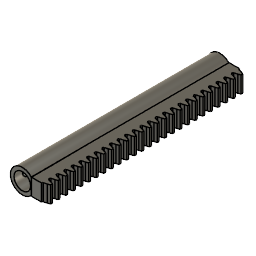
Rack Pen Holder (Autodesk Fusion 360 design; units mm, degrees)
description: Rack; Circular Pitch: 4.12283 mm; Num Teeth: 26; Pressure Angle: 20 deg; Backlash: 0.12 mm;
Autodesk Fusion 360 part; units mm, degrees
note: some values were not read from the file. Set by a fixed rule: which sketch regions a step uses.
(part 1 of 4)
sketch "Sketch1" plane through (0, 0, 0) normal (0, 0, 1) x (1, 0, 0) in component "Rack; Circular Pitch: 4.12283 mm; Num Teeth: 26; Pressure Angle: 20 deg; Backlash: 0.12 mm;"
  line L0 (-1.7283, -1.4496) -> (0, -0.9707)
  line L1 (0, -0.9707) -> (1.3123, -0.4931)
  line L2 (-1.7283, 1.4496) -> (0, 0.9707)
  line L3 (0, 0.9707) -> (1.3123, 0.4931)
  line L4 (1.3123, 0.4931) -> (1.3123, -0.4931)
  line L5 (-2.0948, 1.9315) -> (-2.0948, 2.0614)
  line L6 (-2.0948, -1.9315) -> (-2.0948, -2.0614)
  arc A0 (-2.0948, 1.9315) -> (-1.7283, 1.4496) centre (-1.5948, 1.9315) ccw
  arc A1 (-1.7283, -1.4496) -> (-2.0948, -1.9315) centre (-1.5948, -1.9315) ccw
  line L7 (-1.7283, 2.6732) -> (0, 3.1521)
  line L8 (0, 3.1521) -> (1.3123, 3.6298)
  line L9 (-1.7283, 5.5724) -> (0, 5.0935)
  line L10 (0, 5.0935) -> (1.3123, 4.6159)
  line L11 (1.3123, 4.6159) -> (1.3123, 3.6298)
  line L12 (-2.0948, 6.0543) -> (-2.0948, 6.1842)
  line L13 (-2.0948, 2.1914) -> (-2.0948, 2.0614)
  arc A2 (-2.0948, 6.0543) -> (-1.7283, 5.5724) centre (-1.5948, 6.0543) ccw
  arc A3 (-1.7283, 2.6732) -> (-2.0948, 2.1914) centre (-1.5948, 2.1914) ccw
  line L14 (-1.7283, 6.796) -> (0, 7.275)
  line L15 (0, 7.275) -> (1.3123, 7.7526)
  line L16 (-1.7283, 9.6953) -> (0, 9.2164)
  line L17 (0, 9.2164) -> (1.3123, 8.7387)
  line L18 (1.3123, 8.7387) -> (1.3123, 7.7526)
  line L19 (-2.0948, 10.1771) -> (-2.0948, 10.3071)
  line L20 (-2.0948, 6.3142) -> (-2.0948, 6.1842)
  arc A4 (-2.0948, 10.1771) -> (-1.7283, 9.6953) centre (-1.5948, 10.1771) ccw
  arc A5 (-1.7283, 6.796) -> (-2.0948, 6.3142) centre (-1.5948, 6.3142) ccw
  line L21 (-1.7283, 10.9189) -> (0, 11.3978)
  line L22 (0, 11.3978) -> (1.3123, 11.8754)
  line L23 (-1.7283, 13.8181) -> (0, 13.3392)
  line L24 (0, 13.3392) -> (1.3123, 12.8615)
  line L25 (1.3123, 12.8615) -> (1.3123, 11.8754)
  line L26 (-2.0948, 14.3) -> (-2.0948, 14.4299)
  line L27 (-2.0948, 10.437) -> (-2.0948, 10.3071)
  arc A6 (-2.0948, 14.3) -> (-1.7283, 13.8181) centre (-1.5948, 14.3) ccw
  arc A7 (-1.7283, 10.9189) -> (-2.0948, 10.437) centre (-1.5948, 10.437) ccw
  line L28 (-1.7283, 15.0417) -> (0, 15.5206)
  line L29 (0, 15.5206) -> (1.3123, 15.9983)
  line L30 (-1.7283, 17.9409) -> (0, 17.462)
  line L31 (0, 17.462) -> (1.3123, 16.9844)
  line L32 (1.3123, 16.9844) -> (1.3123, 15.9983)
  line L33 (-2.0948, 18.4228) -> (-2.0948, 18.5527)
  line L34 (-2.0948, 14.5599) -> (-2.0948, 14.4299)
  arc A8 (-2.0948, 18.4228) -> (-1.7283, 17.9409) centre (-1.5948, 18.4228) ccw
  arc A9 (-1.7283, 15.0417) -> (-2.0948, 14.5599) centre (-1.5948, 14.5599) ccw
  line L35 (-1.7283, 19.1645) -> (0, 19.6434)
  line L36 (0, 19.6434) -> (1.3123, 20.1211)
  line L37 (-1.7283, 22.0638) -> (0, 21.5849)
  line L38 (0, 21.5849) -> (1.3123, 21.1072)
  line L39 (1.3123, 21.1072) -> (1.3123, 20.1211)
  line L40 (-2.0948, 22.5456) -> (-2.0948, 22.6756)
  line L41 (-2.0948, 18.6827) -> (-2.0948, 18.5527)
  arc A10 (-2.0948, 22.5456) -> (-1.7283, 22.0638) centre (-1.5948, 22.5456) ccw
  arc A11 (-1.7283, 19.1645) -> (-2.0948, 18.6827) centre (-1.5948, 18.6827) ccw
  line L42 (-1.7283, 23.2874) -> (0, 23.7663)
  line L43 (0, 23.7663) -> (1.3123, 24.2439)
  line L44 (-1.7283, 26.1866) -> (0, 25.7077)
  line L45 (0, 25.7077) -> (1.3123, 25.23)
  line L46 (1.3123, 25.23) -> (1.3123, 24.2439)
  line L47 (-2.0948, 26.6684) -> (-2.0948, 26.7984)
  line L48 (-2.0948, 22.8055) -> (-2.0948, 22.6756)
  arc A12 (-2.0948, 26.6684) -> (-1.7283, 26.1866) centre (-1.5948, 26.6684) ccw
  arc A13 (-1.7283, 23.2874) -> (-2.0948, 22.8055) centre (-1.5948, 22.8055) ccw
  line L49 (-1.7283, 27.4102) -> (0, 27.8891)
  line L50 (0, 27.8891) -> (1.3123, 28.3668)
  line L51 (-1.7283, 30.3094) -> (0, 29.8305)
  line L52 (0, 29.8305) -> (1.3123, 29.3529)
  line L53 (1.3123, 29.3529) -> (1.3123, 28.3668)
  line L54 (-2.0948, 30.7913) -> (-2.0948, 30.9212)
  line L55 (-2.0948, 26.9283) -> (-2.0948, 26.7984)
  arc A14 (-2.0948, 30.7913) -> (-1.7283, 30.3094) centre (-1.5948, 30.7913) ccw
  arc A15 (-1.7283, 27.4102) -> (-2.0948, 26.9283) centre (-1.5948, 26.9283) ccw
  line L56 (-1.7283, 31.533) -> (0, 32.0119)
  line L57 (0, 32.0119) -> (1.3123, 32.4896)
  line L58 (-1.7283, 34.4323) -> (0, 33.9533)
  line L59 (0, 33.9533) -> (1.3123, 33.4757)
  line L60 (1.3123, 33.4757) -> (1.3123, 32.4896)
  line L61 (-2.0948, 34.9141) -> (-2.0948, 35.0441)
  line L62 (-2.0948, 31.0512) -> (-2.0948, 30.9212)
  arc A16 (-2.0948, 34.9141) -> (-1.7283, 34.4323) centre (-1.5948, 34.9141) ccw
  arc A17 (-1.7283, 31.533) -> (-2.0948, 31.0512) centre (-1.5948, 31.0512) ccw
  line L63 (-1.7283, 35.6559) -> (0, 36.1348)
  line L64 (0, 36.1348) -> (1.3123, 36.6124)
  line L65 (-1.7283, 38.5551) -> (0, 38.0762)
  line L66 (0, 38.0762) -> (1.3123, 37.5985)
  line L67 (1.3123, 37.5985) -> (1.3123, 36.6124)
  line L68 (-2.0948, 39.0369) -> (-2.0948, 39.1669)
  line L69 (-2.0948, 35.174) -> (-2.0948, 35.0441)
  arc A18 (-2.0948, 39.0369) -> (-1.7283, 38.5551) centre (-1.5948, 39.0369) ccw
  arc A19 (-1.7283, 35.6559) -> (-2.0948, 35.174) centre (-1.5948, 35.174) ccw
  line L70 (-1.7283, 39.7787) -> (0, 40.2576)
  line L71 (0, 40.2576) -> (1.3123, 40.7352)
  line L72 (-1.7283, 42.6779) -> (0, 42.199)
  line L73 (0, 42.199) -> (1.3123, 41.7214)
  line L74 (1.3123, 41.7214) -> (1.3123, 40.7352)
  line L75 (-2.0948, 43.1598) -> (-2.0948, 43.2897)
  line L76 (-2.0948, 39.2968) -> (-2.0948, 39.1669)
  arc A20 (-2.0948, 43.1598) -> (-1.7283, 42.6779) centre (-1.5948, 43.1598) ccw
  arc A21 (-1.7283, 39.7787) -> (-2.0948, 39.2968) centre (-1.5948, 39.2968) ccw
  line L77 (-1.7283, 43.9015) -> (0, 44.3804)
  line L78 (0, 44.3804) -> (1.3123, 44.8581)
  line L79 (-1.7283, 46.8007) -> (0, 46.3218)
  line L80 (0, 46.3218) -> (1.3123, 45.8442)
  line L81 (1.3123, 45.8442) -> (1.3123, 44.8581)
  line L82 (-2.0948, 47.2826) -> (-2.0948, 47.4125)
  line L83 (-2.0948, 43.4197) -> (-2.0948, 43.2897)
  arc A22 (-2.0948, 47.2826) -> (-1.7283, 46.8007) centre (-1.5948, 47.2826) ccw
  arc A23 (-1.7283, 43.9015) -> (-2.0948, 43.4197) centre (-1.5948, 43.4197) ccw
  line L84 (-1.7283, 48.0243) -> (0, 48.5033)
  line L85 (0, 48.5033) -> (1.3123, 48.9809)
  line L86 (-1.7283, 50.9236) -> (0, 50.4447)
  line L87 (0, 50.4447) -> (1.3123, 49.967)
  line L88 (1.3123, 49.967) -> (1.3123, 48.9809)
  line L89 (-2.0948, 51.4054) -> (-2.0948, 51.5354)
  line L90 (-2.0948, 47.5425) -> (-2.0948, 47.4125)
  arc A24 (-2.0948, 51.4054) -> (-1.7283, 50.9236) centre (-1.5948, 51.4054) ccw
  arc A25 (-1.7283, 48.0243) -> (-2.0948, 47.5425) centre (-1.5948, 47.5425) ccw
  line L91 (-1.7283, 52.1472) -> (0, 52.6261)
  line L92 (0, 52.6261) -> (1.3123, 53.1037)
  line L93 (-1.7283, 55.0464) -> (0, 54.5675)
  line L94 (0, 54.5675) -> (1.3123, 54.0898)
  line L95 (1.3123, 54.0898) -> (1.3123, 53.1037)
  line L96 (-2.0948, 55.5283) -> (-2.0948, 55.6582)
  line L97 (-2.0948, 51.6653) -> (-2.0948, 51.5354)
  arc A26 (-2.0948, 55.5283) -> (-1.7283, 55.0464) centre (-1.5948, 55.5283) ccw
  arc A27 (-1.7283, 52.1472) -> (-2.0948, 51.6653) centre (-1.5948, 51.6653) ccw
  line L98 (-1.7283, 56.27) -> (0, 56.7489)
  line L99 (0, 56.7489) -> (1.3123, 57.2266)
  line L100 (-1.7283, 59.1692) -> (0, 58.6903)
  line L101 (0, 58.6903) -> (1.3123, 58.2127)
  line L102 (1.3123, 58.2127) -> (1.3123, 57.2266)
  line L103 (-2.0948, 59.6511) -> (-2.0948, 59.781)
  line L104 (-2.0948, 55.7882) -> (-2.0948, 55.6582)
  arc A28 (-2.0948, 59.6511) -> (-1.7283, 59.1692) centre (-1.5948, 59.6511) ccw
  arc A29 (-1.7283, 56.27) -> (-2.0948, 55.7882) centre (-1.5948, 55.7882) ccw
  line L105 (-1.7283, 60.3928) -> (0, 60.8717)
  line L106 (0, 60.8717) -> (1.3123, 61.3494)
  line L107 (-1.7283, 63.2921) -> (0, 62.8132)
  line L108 (0, 62.8132) -> (1.3123, 62.3355)
  line L109 (1.3123, 62.3355) -> (1.3123, 61.3494)
  line L110 (-2.0948, 63.7739) -> (-2.0948, 63.9039)
  line L111 (-2.0948, 59.911) -> (-2.0948, 59.781)
  arc A30 (-2.0948, 63.7739) -> (-1.7283, 63.2921) centre (-1.5948, 63.7739) ccw
  arc A31 (-1.7283, 60.3928) -> (-2.0948, 59.911) centre (-1.5948, 59.911) ccw
  line L112 (-1.7283, 64.5157) -> (0, 64.9946)
  line L113 (0, 64.9946) -> (1.3123, 65.4722)
  line L114 (-1.7283, 67.4149) -> (0, 66.936)
  line L115 (0, 66.936) -> (1.3123, 66.4583)
  line L116 (1.3123, 66.4583) -> (1.3123, 65.4722)
  line L117 (-2.0948, 67.8967) -> (-2.0948, 68.0267)
  line L118 (-2.0948, 64.0338) -> (-2.0948, 63.9039)
  arc A32 (-2.0948, 67.8967) -> (-1.7283, 67.4149) centre (-1.5948, 67.8967) ccw
  arc A33 (-1.7283, 64.5157) -> (-2.0948, 64.0338) centre (-1.5948, 64.0338) ccw
  line L119 (-1.7283, 68.6385) -> (0, 69.1174)
  line L120 (0, 69.1174) -> (1.3123, 69.5951)
  line L121 (-1.7283, 71.5377) -> (0, 71.0588)
  line L122 (0, 71.0588) -> (1.3123, 70.5812)
  line L123 (1.3123, 70.5812) -> (1.3123, 69.5951)
  line L124 (-2.0948, 72.0196) -> (-2.0948, 72.1495)
  line L125 (-2.0948, 68.1566) -> (-2.0948, 68.0267)
  arc A34 (-2.0948, 72.0196) -> (-1.7283, 71.5377) centre (-1.5948, 72.0196) ccw
  arc A35 (-1.7283, 68.6385) -> (-2.0948, 68.1566) centre (-1.5948, 68.1566) ccw
  line L126 (-1.7283, 72.7613) -> (0, 73.2402)
  line L127 (0, 73.2402) -> (1.3123, 73.7179)
  line L128 (-1.7283, 75.6606) -> (0, 75.1816)
  line L129 (0, 75.1816) -> (1.3123, 74.704)
  line L130 (1.3123, 74.704) -> (1.3123, 73.7179)
  line L131 (-2.0948, 76.1424) -> (-2.0948, 76.2724)
  line L132 (-2.0948, 72.2795) -> (-2.0948, 72.1495)
  arc A36 (-2.0948, 76.1424) -> (-1.7283, 75.6606) centre (-1.5948, 76.1424) ccw
  arc A37 (-1.7283, 72.7613) -> (-2.0948, 72.2795) centre (-1.5948, 72.2795) ccw
  line L133 (-1.7283, 76.8842) -> (0, 77.3631)
  line L134 (0, 77.3631) -> (1.3123, 77.8407)
  line L135 (-1.7283, 79.7834) -> (0, 79.3045)
  line L136 (0, 79.3045) -> (1.3123, 78.8268)
  line L137 (1.3123, 78.8268) -> (1.3123, 77.8407)
  line L138 (-2.0948, 80.2652) -> (-2.0948, 80.3952)
  line L139 (-2.0948, 76.4023) -> (-2.0948, 76.2724)
  arc A38 (-2.0948, 80.2652) -> (-1.7283, 79.7834) centre (-1.5948, 80.2652) ccw
  arc A39 (-1.7283, 76.8842) -> (-2.0948, 76.4023) centre (-1.5948, 76.4023) ccw
  line L140 (-1.7283, 81.007) -> (0, 81.4859)
  line L141 (0, 81.4859) -> (1.3123, 81.9635)
  line L142 (-1.7283, 83.9062) -> (0, 83.4273)
  line L143 (0, 83.4273) -> (1.3123, 82.9497)
  line L144 (1.3123, 82.9497) -> (1.3123, 81.9635)
  line L145 (-2.0948, 84.3881) -> (-2.0948, 84.518)
  line L146 (-2.0948, 80.5251) -> (-2.0948, 80.3952)
  arc A40 (-2.0948, 84.3881) -> (-1.7283, 83.9062) centre (-1.5948, 84.3881) ccw
  arc A41 (-1.7283, 81.007) -> (-2.0948, 80.5251) centre (-1.5948, 80.5251) ccw
  line L147 (-1.7283, 85.1298) -> (0, 85.6087)
  line L148 (0, 85.6087) -> (1.3123, 86.0864)
  line L149 (-1.7283, 88.029) -> (0, 87.5501)
  line L150 (0, 87.5501) -> (1.3123, 87.0725)
  line L151 (1.3123, 87.0725) -> (1.3123, 86.0864)
  line L152 (-2.0948, 88.5109) -> (-2.0948, 88.6408)
  line L153 (-2.0948, 84.648) -> (-2.0948, 84.518)
  arc A42 (-2.0948, 88.5109) -> (-1.7283, 88.029) centre (-1.5948, 88.5109) ccw
  arc A43 (-1.7283, 85.1298) -> (-2.0948, 84.648) centre (-1.5948, 84.648) ccw
  line L154 (-1.7283, 89.2526) -> (0, 89.7316)
  line L155 (0, 89.7316) -> (1.3123, 90.2092)
  line L156 (-1.7283, 92.1519) -> (0, 91.673)
  line L157 (0, 91.673) -> (1.3123, 91.1953)
  line L158 (1.3123, 91.1953) -> (1.3123, 90.2092)
  line L159 (-2.0948, 92.6337) -> (-2.0948, 92.7637)
  line L160 (-2.0948, 88.7708) -> (-2.0948, 88.6408)
  arc A44 (-2.0948, 92.6337) -> (-1.7283, 92.1519) centre (-1.5948, 92.6337) ccw
  arc A45 (-1.7283, 89.2526) -> (-2.0948, 88.7708) centre (-1.5948, 88.7708) ccw
  line L161 (-1.7283, 93.3755) -> (0, 93.8544)
  line L162 (0, 93.8544) -> (1.3123, 94.332)
  line L163 (-1.7283, 96.2747) -> (0, 95.7958)
  line L164 (0, 95.7958) -> (1.3123, 95.3181)
  line L165 (1.3123, 95.3181) -> (1.3123, 94.332)
  line L166 (-2.0948, 96.7566) -> (-2.0948, 96.8865)
  line L167 (-2.0948, 92.8936) -> (-2.0948, 92.7637)
  arc A46 (-2.0948, 96.7566) -> (-1.7283, 96.2747) centre (-1.5948, 96.7566) ccw
  arc A47 (-1.7283, 93.3755) -> (-2.0948, 92.8936) centre (-1.5948, 92.8936) ccw
  line L168 (-1.7283, 97.4983) -> (0, 97.9772)
  line L169 (0, 97.9772) -> (1.3123, 98.4549)
  line L170 (-1.7283, 100.3975) -> (0, 99.9186)
  line L171 (0, 99.9186) -> (1.3123, 99.441)
  line L172 (1.3123, 99.441) -> (1.3123, 98.4549)
  line L173 (-2.0948, 100.8794) -> (-2.0948, 101.0093)
  line L174 (-2.0948, 97.0165) -> (-2.0948, 96.8865)
  arc A48 (-2.0948, 100.8794) -> (-1.7283, 100.3975) centre (-1.5948, 100.8794) ccw
  arc A49 (-1.7283, 97.4983) -> (-2.0948, 97.0165) centre (-1.5948, 97.0165) ccw
  line L175 (-1.7283, 101.6211) -> (0, 102.1)
  line L176 (0, 102.1) -> (1.3123, 102.5777)
  line L177 (-1.7283, 104.5204) -> (0, 104.0415)
  line L178 (0, 104.0415) -> (1.3123, 103.5638)
  line L179 (1.3123, 103.5638) -> (1.3123, 102.5777)
  line L180 (-2.0948, 105.0022) -> (-2.0948, 105.1322)
  line L181 (-2.0948, 101.1393) -> (-2.0948, 101.0093)
  arc A50 (-2.0948, 105.0022) -> (-1.7283, 104.5204) centre (-1.5948, 105.0022) ccw
  arc A51 (-1.7283, 101.6211) -> (-2.0948, 101.1393) centre (-1.5948, 101.1393) ccw
  line L182 (-1.7283, 105.744) -> (0, 106.2229)
  line L183 (0, 106.2229) -> (1.3123, 106.7005)
  line L184 (-1.7283, 108.6432) -> (0, 108.1643)
  line L185 (0, 108.1643) -> (1.3123, 107.6866)
  line L186 (1.3123, 107.6866) -> (1.3123, 106.7005)
  line L187 (-2.0948, 109.125) -> (-2.0948, 109.255)
  line L188 (-2.0948, 105.2621) -> (-2.0948, 105.1322)
  arc A52 (-2.0948, 109.125) -> (-1.7283, 108.6432) centre (-1.5948, 109.125) ccw
  arc A53 (-1.7283, 105.744) -> (-2.0948, 105.2621) centre (-1.5948, 105.2621) ccw
  line L189 (-2.0948, -2.0614) -> (-7.5948, -2.0614)
  line L190 (-7.5948, -2.0614) -> (-8.0948, 105.1322)
  line L191 (-8.0948, 105.1322) -> (-2.0948, 105.1322)
  constraint tangent L2 A0
  constraint tangent L5 A0
  constraint tangent L0 A1
  constraint tangent L6 A1
  constraint tangent L9 A2
  constraint tangent L12 A2
  constraint tangent L7 A3
  constraint tangent L13 A3
  constraint tangent L16 A4
  constraint tangent L19 A4
  constraint tangent L14 A5
  constraint tangent L20 A5
  constraint tangent L23 A6
  constraint tangent L26 A6
  constraint tangent L21 A7
  constraint tangent L27 A7
  constraint tangent L30 A8
  constraint tangent L33 A8
  constraint tangent L28 A9
  constraint tangent L34 A9
  constraint tangent L37 A10
  constraint tangent L40 A10
  constraint tangent L35 A11
  constraint tangent L41 A11
  constraint tangent L44 A12
  constraint tangent L47 A12
  constraint tangent L42 A13
  constraint tangent L48 A13
  constraint tangent L51 A14
  constraint tangent L54 A14
  constraint tangent L49 A15
  constraint tangent L55 A15
  constraint tangent L58 A16
  constraint tangent L61 A16
  constraint tangent L56 A17
  constraint tangent L62 A17
  constraint tangent L65 A18
  constraint tangent L68 A18
  constraint tangent L63 A19
  constraint tangent L69 A19
  constraint tangent L72 A20
  constraint tangent L75 A20
  constraint tangent L70 A21
  constraint tangent L76 A21
  constraint tangent L79 A22
  constraint tangent L82 A22
  constraint tangent L77 A23
  constraint tangent L83 A23
  constraint tangent L86 A24
  constraint tangent L89 A24
  constraint tangent L84 A25
  constraint tangent L90 A25
  constraint tangent L93 A26
  constraint tangent L96 A26
  constraint tangent L91 A27
  constraint tangent L97 A27
  constraint tangent L100 A28
  constraint tangent L103 A28
  constraint tangent L98 A29
  constraint tangent L104 A29
  constraint tangent L107 A30
  constraint tangent L110 A30
  constraint tangent L105 A31
  constraint tangent L111 A31
  constraint tangent L114 A32
  constraint tangent L117 A32
  constraint tangent L112 A33
  constraint tangent L118 A33
  constraint tangent L121 A34
  constraint tangent L124 A34
  constraint tangent L119 A35
  constraint tangent L125 A35
  constraint tangent L128 A36
  constraint tangent L131 A36
  constraint tangent L126 A37
  constraint tangent L132 A37
  constraint tangent L135 A38
  constraint tangent L138 A38
  constraint tangent L133 A39
  constraint tangent L139 A39
  constraint tangent L142 A40
  constraint tangent L145 A40
  constraint tangent L140 A41
  constraint tangent L146 A41
  constraint tangent L149 A42
  constraint tangent L152 A42
  constraint tangent L147 A43
  constraint tangent L153 A43
  constraint tangent L156 A44
  constraint tangent L159 A44
  constraint tangent L154 A45
  constraint tangent L160 A45
  constraint tangent L163 A46
  constraint tangent L166 A46
  constraint tangent L161 A47
  constraint tangent L167 A47
  constraint tangent L170 A48
  constraint tangent L173 A48
  constraint tangent L168 A49
  constraint tangent L174 A49
  constraint tangent L177 A50
  constraint tangent L180 A50
  constraint tangent L175 A51
  constraint tangent L181 A51
  constraint tangent L184 A52
  constraint tangent L187 A52
  constraint tangent L182 A53
  constraint tangent L188 A53
extrude "Extrude1" add sketch "Sketch1" along normal blind 4.5 and the other way blind 4.5 makes body 1 in component "Rack; Circular Pitch: 4.12283 mm; Num Teeth: 26; Pressure Angle: 20 deg; Backlash: 0.12 mm;"
sketch "Sketch2" plane through (0, 0, 0) normal (0, 0, 1) x (1, 0, 0) in component "Rack; Circular Pitch: 4.12283 mm; Num Teeth: 26; Pressure Angle: 20 deg; Backlash: 0.12 mm;"
  line L0 (0, 0) -> (0, 103.0708) construction
sketch "Sketch1 (2)" plane through (0, 0, 8) normal (0, 0, 1) x (-1, 0, 0)
  arc A0 (-32.6491, -24.8397) -> (-32.7083, -25.327) centre (-17.3506, -26.9445) ccw
  arc A1 (-33.2417, -25.7733) -> (-32.7083, -25.327) centre (-33.2055, -25.2746) ccw
  line L0 (-33.2417, -25.7733) -> (-33.3469, -25.7656)
  spline S0 degree 5 poles (-33.3469, -25.7656) (-33.3537, -25.7652) (-33.3673, -25.7643) (-33.3878, -25.7636) (-33.4151, -25.7635) (-33.4493, -25.7648) (-33.4836, -25.7669) (-33.5178, -25.7697) (-33.5521, -25.7728) (-33.5864, -25.7761) (-33.6207, -25.7796) (-33.655, -25.7834) (-33.6893, -25.7876) (-33.7236, -25.7922) (-33.7579, -25.7974) (-33.7922, -25.8029) (-33.8265, -25.8088) (-33.8609, -25.815) (-33.8952, -25.8214) (-33.9295, -25.8282) (-33.9638, -25.8351) (-33.9981, -25.8424) (-34.0324, -25.8499) (-34.0667, -25.8577) (-34.101, -25.8657) (-34.1353, -25.8741) (-34.1695, -25.8827) (-34.2038, -25.8915) (-34.238, -25.9006) (-34.2723, -25.9099) (-34.3065, -25.9194) (-34.3407, -25.9292) (-34.3749, -25.9392) (-34.4091, -25.9494) (-34.4433, -25.9599) (-34.4775, -25.9706) (-34.5116, -25.9815) (-34.5457, -25.9926) (-34.5799, -26.0039) (-34.614, -26.0154) (-34.6481, -26.0271) (-34.6821, -26.0391) (-34.7162, -26.0512) (-34.7502, -26.0635) (-34.7842, -26.0761) (-34.8182, -26.0888) (-34.8522, -26.1017) (-34.8861, -26.1149) (-34.9201, -26.1282) (-34.954, -26.1417) (-34.9879, -26.1554) (-35.0218, -26.1692) (-35.0556, -26.1833) (-35.0894, -26.1976) (-35.1232, -26.212) (-35.157, -26.2266) (-35.1908, -26.2414) (-35.2245, -26.2564) (-35.2582, -26.2715) (-35.2919, -26.2868) (-35.3256, -26.3023) (-35.3592, -26.318) (-35.3928, -26.3339) (-35.4264, -26.3499) (-35.4599, -26.3661) (-35.4934, -26.3824) (-35.5269, -26.399) (-35.5604, -26.4157) (-35.5938, -26.4325) (-35.6272, -26.4495) (-35.6606, -26.4667) (-35.6873, -26.4806) (-35.7073, -26.4911) (-35.7206, -26.4981) (-35.7273, -26.5017) knots 0 0 0 0 0 0 0.01428571 0.02857143 0.04285714 0.05714286 0.07142857 0.08571429 0.1 0.11428571 0.12857143 0.14285714 0.15714286 0.17142857 0.18571429 0.2 0.21428571 0.22857143 0.24285714 0.25714286 0.27142857 0.28571429 0.3 0.31428571 0.32857143 0.34285714 0.35714286 0.37142857 0.38571429 0.4 0.41428571 0.42857143 0.44285714 0.45714286 0.47142857 0.48571429 0.5 0.51428571 0.52857143 0.54285714 0.55714286 0.57142857 0.58571429 0.6 0.61428571 0.62857143 0.64285714 0.65714286 0.67142857 0.68571429 0.7 0.71428571 0.72857143 0.74285714 0.75714286 0.77142857 0.78571429 0.8 0.81428571 0.82857143 0.84285714 0.85714286 0.87142857 0.88571429 0.9 0.91428571 0.92857143 0.94285714 0.95714286 0.97142857 0.98571429 1 1 1 1 1 1
  arc A2 (-35.7273, -26.5017) -> (-35.7273, -27.3873) centre (-17.3506, -26.9445) ccw
  spline S1 degree 5 poles (-35.7273, -27.3873) (-35.7206, -27.3908) (-35.7073, -27.3979) (-35.6873, -27.4084) (-35.6606, -27.4222) (-35.6272, -27.4394) (-35.5938, -27.4565) (-35.5604, -27.4733) (-35.5269, -27.49) (-35.4934, -27.5066) (-35.4599, -27.5229) (-35.4264, -27.5391) (-35.3928, -27.5551) (-35.3592, -27.571) (-35.3256, -27.5866) (-35.2919, -27.6021) (-35.2582, -27.6175) (-35.2245, -27.6326) (-35.1908, -27.6476) (-35.157, -27.6624) (-35.1232, -27.677) (-35.0894, -27.6914) (-35.0556, -27.7057) (-35.0218, -27.7197) (-34.9879, -27.7336) (-34.954, -27.7473) (-34.9201, -27.7608) (-34.8861, -27.7741) (-34.8522, -27.7872) (-34.8182, -27.8002) (-34.7842, -27.8129) (-34.7502, -27.8254) (-34.7162, -27.8378) (-34.6821, -27.8499) (-34.6481, -27.8618) (-34.614, -27.8736) (-34.5799, -27.8851) (-34.5457, -27.8964) (-34.5116, -27.9075) (-34.4775, -27.9184) (-34.4433, -27.9291) (-34.4091, -27.9395) (-34.3749, -27.9498) (-34.3407, -27.9598) (-34.3065, -27.9695) (-34.2723, -27.9791) (-34.238, -27.9884) (-34.2038, -27.9975) (-34.1695, -28.0063) (-34.1353, -28.0149) (-34.101, -28.0233) (-34.0667, -28.0313) (-34.0324, -28.0391) (-33.9981, -28.0466) (-33.9638, -28.0538) (-33.9295, -28.0608) (-33.8952, -28.0675) (-33.8609, -28.074) (-33.8265, -28.0802) (-33.7922, -28.0861) (-33.7579, -28.0916) (-33.7236, -28.0967) (-33.6893, -28.1014) (-33.655, -28.1056) (-33.6207, -28.1094) (-33.5864, -28.1129) (-33.5521, -28.1162) (-33.5178, -28.1193) (-33.4836, -28.1221) (-33.4493, -28.1242) (-33.4151, -28.1254) (-33.3878, -28.1254) (-33.3673, -28.1247) (-33.3537, -28.1238) (-33.3469, -28.1233) knots -1 -1 -1 -1 -1 -1 -0.98571429 -0.97142857 -0.95714286 -0.94285714 -0.92857143 -0.91428571 -0.9 -0.88571429 -0.87142857 -0.85714286 -0.84285714 -0.82857143 -0.81428571 -0.8 -0.78571429 -0.77142857 -0.75714286 -0.74285714 -0.72857143 -0.71428571 -0.7 -0.68571429 -0.67142857 -0.65714286 -0.64285714 -0.62857143 -0.61428571 -0.6 -0.58571429 -0.57142857 -0.55714286 -0.54285714 -0.52857143 -0.51428571 -0.5 -0.48571429 -0.47142857 -0.45714286 -0.44285714 -0.42857143 -0.41428571 -0.4 -0.38571429 -0.37142857 -0.35714286 -0.34285714 -0.32857143 -0.31428571 -0.3 -0.28571429 -0.27142857 -0.25714286 -0.24285714 -0.22857143 -0.21428571 -0.2 -0.18571429 -0.17142857 -0.15714286 -0.14285714 -0.12857143 -0.11428571 -0.1 -0.08571429 -0.07142857 -0.05714286 -0.04285714 -0.02857143 -0.01428571 0 0 0 0 0 0
  line L1 (-33.3469, -28.1233) -> (-33.2417, -28.1157)
  arc A3 (-32.7083, -28.562) -> (-33.2417, -28.1157) centre (-33.2055, -28.6144) ccw
  arc A4 (-32.7083, -28.562) -> (-32.6491, -29.0493) centre (-17.3506, -26.9445) ccw
  arc A5 (-33.0602, -29.6103) -> (-32.6491, -29.0493) centre (-33.1444, -29.1174) ccw
  line L2 (-33.0602, -29.6103) -> (-33.1641, -29.6281)
  spline S2 degree 5 poles (-33.1641, -29.6281) (-33.1709, -29.6292) (-33.1843, -29.6317) (-33.2044, -29.6358) (-33.231, -29.6423) (-33.2639, -29.6517) (-33.2966, -29.662) (-33.3292, -29.6729) (-33.3617, -29.6841) (-33.3942, -29.6955) (-33.4267, -29.7071) (-33.4591, -29.719) (-33.4914, -29.7313) (-33.5236, -29.744) (-33.5557, -29.7572) (-33.5877, -29.7708) (-33.6196, -29.7847) (-33.6514, -29.799) (-33.6832, -29.8135) (-33.7149, -29.8282) (-33.7465, -29.8432) (-33.7781, -29.8584) (-33.8096, -29.8739) (-33.8411, -29.8897) (-33.8724, -29.9057) (-33.9037, -29.922) (-33.9349, -29.9386) (-33.9661, -29.9553) (-33.9971, -29.9724) (-34.0282, -29.9896) (-34.0591, -30.007) (-34.09, -30.0247) (-34.1208, -30.0426) (-34.1516, -30.0607) (-34.1822, -30.0791) (-34.2129, -30.0976) (-34.2434, -30.1163) (-34.2739, -30.1353) (-34.3043, -30.1544) (-34.3347, -30.1738) (-34.365, -30.1933) (-34.3952, -30.2131) (-34.4253, -30.233) (-34.4554, -30.2531) (-34.4855, -30.2734) (-34.5154, -30.2939) (-34.5453, -30.3146) (-34.5751, -30.3355) (-34.6049, -30.3565) (-34.6346, -30.3778) (-34.6642, -30.3992) (-34.6938, -30.4208) (-34.7233, -30.4425) (-34.7527, -30.4644) (-34.7821, -30.4865) (-34.8114, -30.5088) (-34.8406, -30.5313) (-34.8698, -30.5539) (-34.8989, -30.5766) (-34.9279, -30.5996) (-34.9569, -30.6227) (-34.9858, -30.6459) (-35.0147, -30.6694) (-35.0434, -30.693) (-35.0721, -30.7167) (-35.1008, -30.7406) (-35.1293, -30.7647) (-35.1578, -30.7889) (-35.1862, -30.8133) (-35.2146, -30.8378) (-35.2429, -30.8625) (-35.2655, -30.8824) (-35.2824, -30.8973) (-35.2936, -30.9073) (-35.2993, -30.9124) knots 0 0 0 0 0 0 0.01428571 0.02857143 0.04285714 0.05714286 0.07142857 0.08571429 0.1 0.11428571 0.12857143 0.14285714 0.15714286 0.17142857 0.18571429 0.2 0.21428571 0.22857143 0.24285714 0.25714286 0.27142857 0.28571429 0.3 0.31428571 0.32857143 0.34285714 0.35714286 0.37142857 0.38571429 0.4 0.41428571 0.42857143 0.44285714 0.45714286 0.47142857 0.48571429 0.5 0.51428571 0.52857143 0.54285714 0.55714286 0.57142857 0.58571429 0.6 0.61428571 0.62857143 0.64285714 0.65714286 0.67142857 0.68571429 0.7 0.71428571 0.72857143 0.74285714 0.75714286 0.77142857 0.78571429 0.8 0.81428571 0.82857143 0.84285714 0.85714286 0.87142857 0.88571429 0.9 0.91428571 0.92857143 0.94285714 0.95714286 0.97142857 0.98571429 1 1 1 1 1 1
  arc A6 (-35.2993, -30.9124) -> (-35.0873, -31.7723) centre (-17.3506, -26.9445) ccw
  spline S3 degree 5 poles (-35.0873, -31.7723) (-35.08, -31.7741) (-35.0654, -31.7777) (-35.0435, -31.7831) (-35.0142, -31.7902) (-34.9777, -31.7989) (-34.9412, -31.8075) (-34.9047, -31.8158) (-34.8682, -31.824) (-34.8317, -31.8321) (-34.7953, -31.8399) (-34.7588, -31.8476) (-34.7224, -31.8552) (-34.686, -31.8625) (-34.6496, -31.8697) (-34.6132, -31.8767) (-34.5768, -31.8835) (-34.5404, -31.8901) (-34.5041, -31.8966) (-34.4678, -31.9029) (-34.4315, -31.909) (-34.3952, -31.9149) (-34.359, -31.9206) (-34.3227, -31.9262) (-34.2865, -31.9316) (-34.2504, -31.9367) (-34.2142, -31.9417) (-34.1781, -31.9465) (-34.1419, -31.9512) (-34.1059, -31.9556) (-34.0698, -31.9598) (-34.0338, -31.9638) (-33.9978, -31.9677) (-33.9618, -31.9713) (-33.9259, -31.9747) (-33.89, -31.978) (-33.8541, -31.981) (-33.8183, -31.9838) (-33.7825, -31.9864) (-33.7467, -31.9888) (-33.711, -31.991) (-33.6753, -31.993) (-33.6397, -31.9947) (-33.6041, -31.9963) (-33.5685, -31.9976) (-33.533, -31.9986) (-33.4975, -31.9995) (-33.4621, -32.0001) (-33.4267, -32.0005) (-33.3914, -32.0006) (-33.3561, -32.0005) (-33.3209, -32.0002) (-33.2857, -31.9995) (-33.2506, -31.9986) (-33.2156, -31.9974) (-33.1806, -31.996) (-33.1457, -31.9943) (-33.1108, -31.9923) (-33.076, -31.9902) (-33.0413, -31.9877) (-33.0066, -31.9848) (-32.9721, -31.9816) (-32.9376, -31.9779) (-32.9033, -31.9737) (-32.8691, -31.9692) (-32.835, -31.9644) (-32.8009, -31.9594) (-32.7669, -31.9542) (-32.733, -31.9487) (-32.6992, -31.9426) (-32.6657, -31.9356) (-32.6392, -31.929) (-32.6195, -31.9234) (-32.6064, -31.9193) (-32.5999, -31.9172) knots -1 -1 -1 -1 -1 -1 -0.98571429 -0.97142857 -0.95714286 -0.94285714 -0.92857143 -0.91428571 -0.9 -0.88571429 -0.87142857 -0.85714286 -0.84285714 -0.82857143 -0.81428571 -0.8 -0.78571429 -0.77142857 -0.75714286 -0.74285714 -0.72857143 -0.71428571 -0.7 -0.68571429 -0.67142857 -0.65714286 -0.64285714 -0.62857143 -0.61428571 -0.6 -0.58571429 -0.57142857 -0.55714286 -0.54285714 -0.52857143 -0.51428571 -0.5 -0.48571429 -0.47142857 -0.45714286 -0.44285714 -0.42857143 -0.41428571 -0.4 -0.38571429 -0.37142857 -0.35714286 -0.34285714 -0.32857143 -0.31428571 -0.3 -0.28571429 -0.27142857 -0.25714286 -0.24285714 -0.22857143 -0.21428571 -0.2 -0.18571429 -0.17142857 -0.15714286 -0.14285714 -0.12857143 -0.11428571 -0.1 -0.08571429 -0.07142857 -0.05714286 -0.04285714 -0.02857143 -0.01428571 0 0 0 0 0 0
  line L3 (-32.5999, -31.9172) -> (-32.4996, -31.8847)
  arc A7 (-31.8749, -32.1904) -> (-32.4996, -31.8847) centre (-32.3452, -32.3602) ccw
  arc A8 (-31.8749, -32.1904) -> (-31.7009, -32.6493) centre (-17.3506, -26.9445) ccw
  arc A9 (-31.9657, -33.2924) -> (-31.7009, -32.6493) centre (-32.1655, -32.834) ccw
  line L4 (-31.9657, -33.2924) -> (-32.0624, -33.3345)
  spline S4 degree 5 poles (-32.0624, -33.3345) (-32.0687, -33.3372) (-32.0812, -33.3428) (-32.0996, -33.3517) (-32.1239, -33.3644) (-32.1536, -33.3813) (-32.1829, -33.3992) (-32.2119, -33.4175) (-32.2408, -33.4362) (-32.2697, -33.455) (-32.2984, -33.4741) (-32.327, -33.4934) (-32.3554, -33.5131) (-32.3836, -33.5331) (-32.4117, -33.5536) (-32.4395, -33.5744) (-32.4671, -33.5956) (-32.4946, -33.617) (-32.522, -33.6387) (-32.5493, -33.6606) (-32.5764, -33.6827) (-32.6034, -33.7051) (-32.6303, -33.7277) (-32.657, -33.7505) (-32.6837, -33.7736) (-32.7101, -33.7969) (-32.7365, -33.8204) (-32.7627, -33.8442) (-32.7888, -33.8681) (-32.8148, -33.8923) (-32.8407, -33.9167) (-32.8664, -33.9412) (-32.8921, -33.966) (-32.9176, -33.9909) (-32.943, -34.016) (-32.9683, -34.0414) (-32.9935, -34.0669) (-33.0185, -34.0926) (-33.0435, -34.1185) (-33.0683, -34.1445) (-33.0931, -34.1707) (-33.1177, -34.1971) (-33.1422, -34.2237) (-33.1666, -34.2504) (-33.1909, -34.2773) (-33.2151, -34.3044) (-33.2391, -34.3317) (-33.2631, -34.3591) (-33.287, -34.3866) (-33.3107, -34.4143) (-33.3344, -34.4422) (-33.3579, -34.4702) (-33.3814, -34.4984) (-33.4047, -34.5268) (-33.4279, -34.5552) (-33.451, -34.5839) (-33.474, -34.6127) (-33.497, -34.6416) (-33.5198, -34.6707) (-33.5425, -34.6999) (-33.5651, -34.7293) (-33.5876, -34.7588) (-33.6099, -34.7884) (-33.6322, -34.8182) (-33.6544, -34.8481) (-33.6765, -34.8782) (-33.6985, -34.9084) (-33.7203, -34.9387) (-33.7421, -34.9692) (-33.7638, -34.9998) (-33.7853, -35.0305) (-33.8025, -35.0552) (-33.8153, -35.0738) (-33.8239, -35.0862) (-33.8281, -35.0924) knots 0 0 0 0 0 0 0.01428571 0.02857143 0.04285714 0.05714286 0.07142857 0.08571429 0.1 0.11428571 0.12857143 0.14285714 0.15714286 0.17142857 0.18571429 0.2 0.21428571 0.22857143 0.24285714 0.25714286 0.27142857 0.28571429 0.3 0.31428571 0.32857143 0.34285714 0.35714286 0.37142857 0.38571429 0.4 0.41428571 0.42857143 0.44285714 0.45714286 0.47142857 0.48571429 0.5 0.51428571 0.52857143 0.54285714 0.55714286 0.57142857 0.58571429 0.6 0.61428571 0.62857143 0.64285714 0.65714286 0.67142857 0.68571429 0.7 0.71428571 0.72857143 0.74285714 0.75714286 0.77142857 0.78571429 0.8 0.81428571 0.82857143 0.84285714 0.85714286 0.87142857 0.88571429 0.9 0.91428571 0.92857143 0.94285714 0.95714286 0.97142857 0.98571429 1 1 1 1 1 1
  arc A10 (-33.8281, -35.0924) -> (-33.4166, -35.8767) centre (-17.3506, -26.9445) ccw
  spline S5 degree 5 poles (-33.4166, -35.8767) (-33.409, -35.8767) (-33.394, -35.8767) (-33.3714, -35.8767) (-33.3413, -35.8766) (-33.3038, -35.8763) (-33.2663, -35.8759) (-33.2288, -35.8753) (-33.1914, -35.8745) (-33.1541, -35.8736) (-33.1168, -35.8725) (-33.0796, -35.8712) (-33.0424, -35.8698) (-33.0053, -35.8682) (-32.9682, -35.8665) (-32.9312, -35.8645) (-32.8943, -35.8625) (-32.8574, -35.8602) (-32.8206, -35.8578) (-32.7838, -35.8552) (-32.7471, -35.8524) (-32.7104, -35.8495) (-32.6739, -35.8464) (-32.6374, -35.8431) (-32.6009, -35.8397) (-32.5646, -35.836) (-32.5282, -35.8322) (-32.492, -35.8283) (-32.4558, -35.8241) (-32.4198, -35.8198) (-32.3837, -35.8152) (-32.3478, -35.8105) (-32.3119, -35.8056) (-32.2761, -35.8006) (-32.2404, -35.7953) (-32.2048, -35.7898) (-32.1692, -35.7842) (-32.1338, -35.7783) (-32.0984, -35.7723) (-32.0631, -35.7661) (-32.0279, -35.7597) (-31.9928, -35.753) (-31.9577, -35.7462) (-31.9228, -35.7392) (-31.888, -35.7319) (-31.8532, -35.7245) (-31.8186, -35.7168) (-31.784, -35.7089) (-31.7496, -35.7008) (-31.7152, -35.6925) (-31.681, -35.684) (-31.6469, -35.6752) (-31.6129, -35.6661) (-31.5791, -35.6568) (-31.5453, -35.6473) (-31.5117, -35.6375) (-31.4782, -35.6275) (-31.4448, -35.6173) (-31.4115, -35.6069) (-31.3784, -35.5961) (-31.3455, -35.5851) (-31.3127, -35.5736) (-31.2802, -35.5618) (-31.2478, -35.5496) (-31.2157, -35.537) (-31.1837, -35.5242) (-31.1518, -35.5112) (-31.12, -35.498) (-31.0884, -35.4845) (-31.0571, -35.4705) (-31.0262, -35.4557) (-31.002, -35.443) (-30.9843, -35.4328) (-30.9726, -35.4257) (-30.9667, -35.4221) knots -1 -1 -1 -1 -1 -1 -0.98571429 -0.97142857 -0.95714286 -0.94285714 -0.92857143 -0.91428571 -0.9 -0.88571429 -0.87142857 -0.85714286 -0.84285714 -0.82857143 -0.81428571 -0.8 -0.78571429 -0.77142857 -0.75714286 -0.74285714 -0.72857143 -0.71428571 -0.7 -0.68571429 -0.67142857 -0.65714286 -0.64285714 -0.62857143 -0.61428571 -0.6 -0.58571429 -0.57142857 -0.55714286 -0.54285714 -0.52857143 -0.51428571 -0.5 -0.48571429 -0.47142857 -0.45714286 -0.44285714 -0.42857143 -0.41428571 -0.4 -0.38571429 -0.37142857 -0.35714286 -0.34285714 -0.32857143 -0.31428571 -0.3 -0.28571429 -0.27142857 -0.25714286 -0.24285714 -0.22857143 -0.21428571 -0.2 -0.18571429 -0.17142857 -0.15714286 -0.14285714 -0.12857143 -0.11428571 -0.1 -0.08571429 -0.07142857 -0.05714286 -0.04285714 -0.02857143 -0.01428571 0 0 0 0 0 0
  line L5 (-30.9667, -35.4221) -> (-30.8771, -35.3665)
  arc A11 (-30.1974, -35.5138) -> (-30.8771, -35.3665) centre (-30.6134, -35.7913) ccw
  arc A12 (-30.1974, -35.5138) -> (-29.9186, -35.9178) centre (-17.3506, -26.9445) ccw
  arc A13 (-30.0219, -36.6055) -> (-29.9186, -35.9178) centre (-30.3255, -36.2083) ccw
  line L6 (-30.0219, -36.6055) -> (-30.1057, -36.6696)
  spline S6 degree 5 poles (-30.1057, -36.6696) (-30.1111, -36.6737) (-30.1219, -36.6822) (-30.1377, -36.6952) (-30.1582, -36.7133) (-30.183, -36.7369) (-30.2072, -36.7612) (-30.231, -36.786) (-30.2546, -36.811) (-30.2781, -36.8362) (-30.3014, -36.8616) (-30.3245, -36.8872) (-30.3474, -36.9131) (-30.37, -36.9393) (-30.3923, -36.9659) (-30.4144, -36.9928) (-30.4361, -37.02) (-30.4577, -37.0474) (-30.4791, -37.075) (-30.5003, -37.1027) (-30.5214, -37.1307) (-30.5423, -37.1589) (-30.563, -37.1872) (-30.5835, -37.2158) (-30.6038, -37.2446) (-30.6239, -37.2735) (-30.6439, -37.3027) (-30.6637, -37.332) (-30.6833, -37.3616) (-30.7027, -37.3912) (-30.722, -37.4211) (-30.7411, -37.4511) (-30.7601, -37.4812) (-30.7789, -37.5116) (-30.7976, -37.5421) (-30.8161, -37.5727) (-30.8344, -37.6035) (-30.8526, -37.6344) (-30.8706, -37.6655) (-30.8885, -37.6968) (-30.9063, -37.7282) (-30.9238, -37.7597) (-30.9413, -37.7913) (-30.9586, -37.8232) (-30.9757, -37.8551) (-30.9927, -37.8872) (-31.0096, -37.9194) (-31.0263, -37.9517) (-31.0429, -37.9842) (-31.0593, -38.0168) (-31.0756, -38.0495) (-31.0917, -38.0823) (-31.1078, -38.1153) (-31.1236, -38.1484) (-31.1394, -38.1816) (-31.155, -38.215) (-31.1704, -38.2484) (-31.1857, -38.282) (-31.2009, -38.3157) (-31.216, -38.3495) (-31.2309, -38.3834) (-31.2457, -38.4175) (-31.2603, -38.4516) (-31.2748, -38.4859) (-31.2892, -38.5202) (-31.3034, -38.5547) (-31.3175, -38.5893) (-31.3315, -38.624) (-31.3454, -38.6588) (-31.3591, -38.6937) (-31.3727, -38.7287) (-31.3834, -38.7568) (-31.3914, -38.7779) (-31.3967, -38.792) (-31.3994, -38.799) knots 0 0 0 0 0 0 0.01428571 0.02857143 0.04285714 0.05714286 0.07142857 0.08571429 0.1 0.11428571 0.12857143 0.14285714 0.15714286 0.17142857 0.18571429 0.2 0.21428571 0.22857143 0.24285714 0.25714286 0.27142857 0.28571429 0.3 0.31428571 0.32857143 0.34285714 0.35714286 0.37142857 0.38571429 0.4 0.41428571 0.42857143 0.44285714 0.45714286 0.47142857 0.48571429 0.5 0.51428571 0.52857143 0.54285714 0.55714286 0.57142857 0.58571429 0.6 0.61428571 0.62857143 0.64285714 0.65714286 0.67142857 0.68571429 0.7 0.71428571 0.72857143 0.74285714 0.75714286 0.77142857 0.78571429 0.8 0.81428571 0.82857143 0.84285714 0.85714286 0.87142857 0.88571429 0.9 0.91428571 0.92857143 0.94285714 0.95714286 0.97142857 0.98571429 1 1 1 1 1 1
  arc A14 (-31.3994, -38.799) -> (-30.8121, -39.4619) centre (-17.3506, -26.9445) ccw
  spline S7 degree 5 poles (-30.8121, -39.4619) (-30.8048, -39.4602) (-30.7901, -39.4566) (-30.7682, -39.4512) (-30.739, -39.4439) (-30.7027, -39.4346) (-30.6664, -39.4252) (-30.6302, -39.4156) (-30.594, -39.406) (-30.558, -39.3961) (-30.5221, -39.3861) (-30.4862, -39.376) (-30.4505, -39.3657) (-30.4148, -39.3553) (-30.3792, -39.3447) (-30.3438, -39.334) (-30.3084, -39.3232) (-30.2731, -39.3121) (-30.2379, -39.301) (-30.2029, -39.2897) (-30.1679, -39.2782) (-30.133, -39.2666) (-30.0982, -39.2548) (-30.0636, -39.2429) (-30.029, -39.2308) (-29.9946, -39.2186) (-29.9602, -39.2062) (-29.926, -39.1937) (-29.8919, -39.181) (-29.8579, -39.1681) (-29.824, -39.1551) (-29.7902, -39.142) (-29.7566, -39.1286) (-29.723, -39.1151) (-29.6896, -39.1015) (-29.6563, -39.0876) (-29.6232, -39.0736) (-29.5901, -39.0595) (-29.5572, -39.0452) (-29.5244, -39.0307) (-29.4918, -39.016) (-29.4593, -39.0012) (-29.4269, -38.9862) (-29.3946, -38.971) (-29.3626, -38.9556) (-29.3306, -38.94) (-29.2988, -38.9243) (-29.2671, -38.9084) (-29.2356, -38.8923) (-29.2043, -38.876) (-29.1731, -38.8595) (-29.1421, -38.8428) (-29.1112, -38.8259) (-29.0806, -38.8088) (-29.0501, -38.7914) (-29.0198, -38.7739) (-28.9897, -38.7562) (-28.9597, -38.7383) (-28.9299, -38.7201) (-28.9003, -38.7018) (-28.871, -38.6832) (-28.8419, -38.6642) (-28.8131, -38.645) (-28.7847, -38.6254) (-28.7564, -38.6055) (-28.7284, -38.5854) (-28.7006, -38.5651) (-28.6729, -38.5447) (-28.6454, -38.524) (-28.6184, -38.503) (-28.592, -38.4812) (-28.5715, -38.463) (-28.5567, -38.4489) (-28.547, -38.4392) (-28.5423, -38.4343) knots -1 -1 -1 -1 -1 -1 -0.98571429 -0.97142857 -0.95714286 -0.94285714 -0.92857143 -0.91428571 -0.9 -0.88571429 -0.87142857 -0.85714286 -0.84285714 -0.82857143 -0.81428571 -0.8 -0.78571429 -0.77142857 -0.75714286 -0.74285714 -0.72857143 -0.71428571 -0.7 -0.68571429 -0.67142857 -0.65714286 -0.64285714 -0.62857143 -0.61428571 -0.6 -0.58571429 -0.57142857 -0.55714286 -0.54285714 -0.52857143 -0.51428571 -0.5 -0.48571429 -0.47142857 -0.45714286 -0.44285714 -0.42857143 -0.41428571 -0.4 -0.38571429 -0.37142857 -0.35714286 -0.34285714 -0.32857143 -0.31428571 -0.3 -0.28571429 -0.27142857 -0.25714286 -0.24285714 -0.22857143 -0.21428571 -0.2 -0.18571429 -0.17142857 -0.15714286 -0.14285714 -0.12857143 -0.11428571 -0.1 -0.08571429 -0.07142857 -0.05714286 -0.04285714 -0.02857143 -0.01428571 0 0 0 0 0 0
  line L7 (-28.5423, -38.4343) -> (-28.4686, -38.3589)
  arc A15 (-27.7734, -38.3392) -> (-28.4686, -38.3589) centre (-28.1108, -38.7082) ccw
  arc A16 (-27.7734, -38.3392) -> (-27.406, -38.6647) centre (-17.3506, -26.9445) ccw
  arc A17 (-27.3417, -39.3572) -> (-27.406, -38.6647) centre (-27.7315, -39.0442) ccw
  line L8 (-27.3417, -39.3572) -> (-27.4077, -39.4395)
  spline S8 degree 5 poles (-27.4077, -39.4395) (-27.412, -39.4448) (-27.4204, -39.4556) (-27.4326, -39.472) (-27.4482, -39.4945) (-27.4666, -39.5233) (-27.4843, -39.5527) (-27.5015, -39.5825) (-27.5184, -39.6124) (-27.5352, -39.6425) (-27.5518, -39.6727) (-27.5681, -39.7031) (-27.5841, -39.7338) (-27.5998, -39.7646) (-27.6151, -39.7958) (-27.63, -39.8272) (-27.6447, -39.8588) (-27.6591, -39.8905) (-27.6732, -39.9224) (-27.6872, -39.9545) (-27.701, -39.9867) (-27.7145, -40.019) (-27.7278, -40.0515) (-27.7409, -40.0842) (-27.7537, -40.117) (-27.7663, -40.1499) (-27.7787, -40.183) (-27.7909, -40.2162) (-27.8029, -40.2496) (-27.8147, -40.283) (-27.8263, -40.3166) (-27.8377, -40.3503) (-27.8489, -40.3842) (-27.8599, -40.4181) (-27.8707, -40.4522) (-27.8813, -40.4864) (-27.8917, -40.5206) (-27.902, -40.555) (-27.9121, -40.5896) (-27.9219, -40.6242) (-27.9317, -40.6589) (-27.9412, -40.6937) (-27.9505, -40.7286) (-27.9597, -40.7636) (-27.9687, -40.7987) (-27.9776, -40.834) (-27.9862, -40.8693) (-27.9947, -40.9047) (-28.003, -40.9402) (-28.0112, -40.9757) (-28.0192, -41.0114) (-28.027, -41.0472) (-28.0346, -41.083) (-28.0421, -41.1189) (-28.0495, -41.155) (-28.0566, -41.1911) (-28.0636, -41.2272) (-28.0705, -41.2635) (-28.0771, -41.2999) (-28.0837, -41.3363) (-28.09, -41.3728) (-28.0962, -41.4094) (-28.1023, -41.446) (-28.1082, -41.4828) (-28.1139, -41.5196) (-28.1195, -41.5565) (-28.1249, -41.5934) (-28.1302, -41.6304) (-28.1353, -41.6675) (-28.1403, -41.7047) (-28.1451, -41.7419) (-28.1488, -41.7718) (-28.1515, -41.7942) (-28.1533, -41.8092) (-28.1542, -41.8166) knots 0 0 0 0 0 0 0.01428571 0.02857143 0.04285714 0.05714286 0.07142857 0.08571429 0.1 0.11428571 0.12857143 0.14285714 0.15714286 0.17142857 0.18571429 0.2 0.21428571 0.22857143 0.24285714 0.25714286 0.27142857 0.28571429 0.3 0.31428571 0.32857143 0.34285714 0.35714286 0.37142857 0.38571429 0.4 0.41428571 0.42857143 0.44285714 0.45714286 0.47142857 0.48571429 0.5 0.51428571 0.52857143 0.54285714 0.55714286 0.57142857 0.58571429 0.6 0.61428571 0.62857143 0.64285714 0.65714286 0.67142857 0.68571429 0.7 0.71428571 0.72857143 0.74285714 0.75714286 0.77142857 0.78571429 0.8 0.81428571 0.82857143 0.84285714 0.85714286 0.87142857 0.88571429 0.9 0.91428571 0.92857143 0.94285714 0.95714286 0.97142857 0.98571429 1 1 1 1 1 1
  arc A18 (-28.1542, -41.8166) -> (-27.4253, -42.3197) centre (-17.3506, -26.9445) ccw
  spline S9 degree 5 poles (-27.4253, -42.3197) (-27.4186, -42.3163) (-27.4053, -42.3093) (-27.3853, -42.2988) (-27.3587, -42.2847) (-27.3256, -42.267) (-27.2926, -42.2492) (-27.2597, -42.2313) (-27.227, -42.2132) (-27.1943, -42.195) (-27.1618, -42.1767) (-27.1295, -42.1583) (-27.0972, -42.1398) (-27.0651, -42.1211) (-27.0331, -42.1024) (-27.0012, -42.0835) (-26.9694, -42.0645) (-26.9378, -42.0453) (-26.9063, -42.0261) (-26.875, -42.0067) (-26.8438, -41.9872) (-26.8127, -41.9676) (-26.7818, -41.9478) (-26.751, -41.9279) (-26.7203, -41.908) (-26.6898, -41.8878) (-26.6594, -41.8676) (-26.6292, -41.8472) (-26.5991, -41.8267) (-26.5691, -41.8061) (-26.5393, -41.7854) (-26.5097, -41.7645) (-26.4802, -41.7435) (-26.4509, -41.7224) (-26.4217, -41.7011) (-26.3927, -41.6797) (-26.3638, -41.6582) (-26.3351, -41.6366) (-26.3066, -41.6148) (-26.2783, -41.5929) (-26.2501, -41.5708) (-26.222, -41.5486) (-26.1942, -41.5263) (-26.1665, -41.5038) (-26.1391, -41.4812) (-26.1118, -41.4585) (-26.0847, -41.4356) (-26.0577, -41.4125) (-26.031, -41.3894) (-26.0044, -41.366) (-25.9781, -41.3426) (-25.952, -41.3189) (-25.9261, -41.2951) (-25.9004, -41.2712) (-25.875, -41.2471) (-25.8498, -41.2228) (-25.8248, -41.1984) (-25.7999, -41.1738) (-25.7753, -41.1491) (-25.751, -41.1242) (-25.7269, -41.0991) (-25.7033, -41.0737) (-25.6799, -41.0481) (-25.657, -41.0223) (-25.6344, -40.9962) (-25.612, -40.97) (-25.5898, -40.9437) (-25.5678, -40.9172) (-25.5461, -40.8906) (-25.5248, -40.8636) (-25.5044, -40.8362) (-25.4889, -40.8137) (-25.4779, -40.7964) (-25.4708, -40.7847) (-25.4673, -40.7788) knots -1 -1 -1 -1 -1 -1 -0.98571429 -0.97142857 -0.95714286 -0.94285714 -0.92857143 -0.91428571 -0.9 -0.88571429 -0.87142857 -0.85714286 -0.84285714 -0.82857143 -0.81428571 -0.8 -0.78571429 -0.77142857 -0.75714286 -0.74285714 -0.72857143 -0.71428571 -0.7 -0.68571429 -0.67142857 -0.65714286 -0.64285714 -0.62857143 -0.61428571 -0.6 -0.58571429 -0.57142857 -0.55714286 -0.54285714 -0.52857143 -0.51428571 -0.5 -0.48571429 -0.47142857 -0.45714286 -0.44285714 -0.42857143 -0.41428571 -0.4 -0.38571429 -0.37142857 -0.35714286 -0.34285714 -0.32857143 -0.31428571 -0.3 -0.28571429 -0.27142857 -0.25714286 -0.24285714 -0.22857143 -0.21428571 -0.2 -0.18571429 -0.17142857 -0.15714286 -0.14285714 -0.12857143 -0.11428571 -0.1 -0.08571429 -0.07142857 -0.05714286 -0.04285714 -0.02857143 -0.01428571 0 0 0 0 0 0
  line L9 (-25.4673, -40.7788) -> (-25.4139, -40.6879)
  arc A19 (-24.7436, -40.5025) -> (-25.4139, -40.6879) centre (-24.9829, -40.9414) ccw
  arc A20 (-24.7436, -40.5025) -> (-24.3089, -40.7306) centre (-17.3506, -26.9445) ccw
  arc A21 (-24.0808, -41.3876) -> (-24.3089, -40.7306) centre (-24.5342, -41.1769) ccw
  line L10 (-24.0808, -41.3876) -> (-24.1252, -41.4832)
  spline S10 degree 5 poles (-24.1252, -41.4832) (-24.1281, -41.4894) (-24.1337, -41.5019) (-24.1416, -41.5208) (-24.1514, -41.5463) (-24.1624, -41.5787) (-24.1725, -41.6115) (-24.1821, -41.6445) (-24.1913, -41.6776) (-24.2004, -41.7108) (-24.2093, -41.7442) (-24.2179, -41.7776) (-24.2261, -41.8112) (-24.2339, -41.8449) (-24.2413, -41.8788) (-24.2483, -41.9128) (-24.255, -41.947) (-24.2613, -41.9813) (-24.2675, -42.0157) (-24.2734, -42.0502) (-24.279, -42.0847) (-24.2844, -42.1193) (-24.2896, -42.1541) (-24.2944, -42.1889) (-24.299, -42.2238) (-24.3034, -42.2588) (-24.3075, -42.2939) (-24.3114, -42.3291) (-24.315, -42.3643) (-24.3185, -42.3996) (-24.3217, -42.435) (-24.3247, -42.4705) (-24.3275, -42.506) (-24.33, -42.5416) (-24.3324, -42.5773) (-24.3345, -42.613) (-24.3364, -42.6488) (-24.3382, -42.6847) (-24.3397, -42.7206) (-24.341, -42.7565) (-24.3421, -42.7926) (-24.343, -42.8287) (-24.3438, -42.8648) (-24.3443, -42.901) (-24.3446, -42.9372) (-24.3448, -42.9735) (-24.3447, -43.0099) (-24.3445, -43.0463) (-24.3441, -43.0828) (-24.3435, -43.1193) (-24.3427, -43.1558) (-24.3418, -43.1924) (-24.3406, -43.229) (-24.3393, -43.2657) (-24.3378, -43.3024) (-24.3361, -43.3392) (-24.3342, -43.376) (-24.3322, -43.4129) (-24.33, -43.4497) (-24.3276, -43.4867) (-24.325, -43.5236) (-24.3223, -43.5606) (-24.3194, -43.5977) (-24.3163, -43.6348) (-24.3131, -43.6719) (-24.3097, -43.709) (-24.3061, -43.7462) (-24.3024, -43.7834) (-24.2985, -43.8206) (-24.2944, -43.8579) (-24.2901, -43.8952) (-24.2866, -43.9251) (-24.2839, -43.9475) (-24.2821, -43.9625) (-24.2811, -43.9699) knots 0 0 0 0 0 0 0.01428571 0.02857143 0.04285714 0.05714286 0.07142857 0.08571429 0.1 0.11428571 0.12857143 0.14285714 0.15714286 0.17142857 0.18571429 0.2 0.21428571 0.22857143 0.24285714 0.25714286 0.27142857 0.28571429 0.3 0.31428571 0.32857143 0.34285714 0.35714286 0.37142857 0.38571429 0.4 0.41428571 0.42857143 0.44285714 0.45714286 0.47142857 0.48571429 0.5 0.51428571 0.52857143 0.54285714 0.55714286 0.57142857 0.58571429 0.6 0.61428571 0.62857143 0.64285714 0.65714286 0.67142857 0.68571429 0.7 0.71428571 0.72857143 0.74285714 0.75714286 0.77142857 0.78571429 0.8 0.81428571 0.82857143 0.84285714 0.85714286 0.87142857 0.88571429 0.9 0.91428571 0.92857143 0.94285714 0.95714286 0.97142857 0.98571429 1 1 1 1 1 1
  arc A22 (-24.2811, -43.9699) -> (-23.453, -44.284) centre (-17.3506, -26.9445) ccw
  spline S11 degree 5 poles (-23.453, -44.284) (-23.4474, -44.279) (-23.4361, -44.2691) (-23.4192, -44.2541) (-23.3967, -44.2341) (-23.3688, -44.2089) (-23.341, -44.1837) (-23.3134, -44.1585) (-23.2859, -44.1331) (-23.2586, -44.1076) (-23.2314, -44.0821) (-23.2044, -44.0565) (-23.1775, -44.0307) (-23.1508, -44.0049) (-23.1242, -43.9791) (-23.0978, -43.9531) (-23.0715, -43.927) (-23.0454, -43.9009) (-23.0194, -43.8747) (-22.9936, -43.8483) (-22.968, -43.8219) (-22.9425, -43.7954) (-22.9172, -43.7689) (-22.892, -43.7422) (-22.867, -43.7155) (-22.8422, -43.6886) (-22.8176, -43.6617) (-22.7931, -43.6347) (-22.7688, -43.6076) (-22.7446, -43.5804) (-22.7207, -43.5531) (-22.6969, -43.5258) (-22.6733, -43.4983) (-22.6499, -43.4708) (-22.6266, -43.4432) (-22.6036, -43.4155) (-22.5807, -43.3877) (-22.558, -43.3598) (-22.5355, -43.3318) (-22.5132, -43.3037) (-22.4912, -43.2756) (-22.4693, -43.2473) (-22.4476, -43.219) (-22.4261, -43.1905) (-22.4048, -43.162) (-22.3838, -43.1334) (-22.3629, -43.1047) (-22.3423, -43.0759) (-22.3219, -43.047) (-22.3017, -43.018) (-22.2817, -42.9889) (-22.262, -42.9597) (-22.2426, -42.9304) (-22.2234, -42.901) (-22.2045, -42.8715) (-22.1858, -42.8419) (-22.1673, -42.8122) (-22.1491, -42.7824) (-22.1312, -42.7525) (-22.1135, -42.7225) (-22.0961, -42.6924) (-22.0792, -42.6621) (-22.0627, -42.6316) (-22.0466, -42.6011) (-22.0308, -42.5703) (-22.0154, -42.5395) (-22.0001, -42.5086) (-21.9851, -42.4777) (-21.9704, -42.4466) (-21.9562, -42.4154) (-21.943, -42.3838) (-21.9333, -42.3583) (-21.9267, -42.3389) (-21.9227, -42.3258) (-21.9207, -42.3193) knots -1 -1 -1 -1 -1 -1 -0.98571429 -0.97142857 -0.95714286 -0.94285714 -0.92857143 -0.91428571 -0.9 -0.88571429 -0.87142857 -0.85714286 -0.84285714 -0.82857143 -0.81428571 -0.8 -0.78571429 -0.77142857 -0.75714286 -0.74285714 -0.72857143 -0.71428571 -0.7 -0.68571429 -0.67142857 -0.65714286 -0.64285714 -0.62857143 -0.61428571 -0.6 -0.58571429 -0.57142857 -0.55714286 -0.54285714 -0.52857143 -0.51428571 -0.5 -0.48571429 -0.47142857 -0.45714286 -0.44285714 -0.42857143 -0.41428571 -0.4 -0.38571429 -0.37142857 -0.35714286 -0.34285714 -0.32857143 -0.31428571 -0.3 -0.28571429 -0.27142857 -0.25714286 -0.24285714 -0.22857143 -0.21428571 -0.2 -0.18571429 -0.17142857 -0.15714286 -0.14285714 -0.12857143 -0.11428571 -0.1 -0.08571429 -0.07142857 -0.05714286 -0.04285714 -0.02857143 -0.01428571 0 0 0 0 0 0
  line L11 (-21.9207, -42.3193) -> (-21.8906, -42.2182)
  arc A23 (-21.2841, -41.8777) -> (-21.8906, -42.2182) centre (-21.4115, -42.3612) ccw
  arc A24 (-21.2841, -41.8777) -> (-20.8075, -41.9952) centre (-17.3506, -26.9445) ccw
  arc A25 (-20.4288, -42.5785) -> (-20.8075, -41.9952) centre (-20.9195, -42.4825) ccw
  line L12 (-20.4288, -42.5785) -> (-20.449, -42.682)